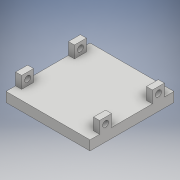
# Autodesk Inventor part: steven_example
Saved by Autodesk Inventor 2018 (Build 220112000, 112)
## iProperties
Created: 2018-03-21
Part Number: steven_example
Material: Generic
Document SubType Name: Modeling
Designer: dvyen
Density: 1 g/cm^3
Appearance: Default
Author: dvyen
Autodesk Inventor part; units mm, degrees
ref_plane "YZ Plane" through (0, 0, 0) normal (1, 0, 0) x (0, 1, 0)
ref_plane "XZ Plane" through (0, 0, 0) normal (0, 1, 0) x (-1, 0, 0)
ref_plane "XY Plane" through (0, 0, 0) normal (0, 0, 1) x (1, 0, 0)
sketch "Sketch1" plane through (0, 0, 0) normal (0, 0, 1) x (1, 0, 0)
  line L0 (-35, 35) -> (35, 35)
  line L1 (35, 35) -> (35, -35)
  line L2 (35, -35) -> (-35, -35)
  line L3 (-35, -35) -> (-35, 35)
  point P0 (0, 0)
  dimension "d0" = 70
  dimension "d1" = 70
  dimension "d2" = 35
  dimension "d3" = 35
  constraints: 8 end point, 2 parallel, 1 horizontal, 1 perpendicular
  measures "d0" distance of L0.start L0.end
  measures "d1" distance of L2.end L0.start
  measures "d2" distance from line of point (0, 0) L3
  measures "d3" distance from line of point (0, 0) L0
extrude "Extrusion1" add sketch "Sketch1" along normal blind 8
sketch "Sketch2" plane through (0, 0, 8) normal (0, 0, 1) x (1, 0, 0)
  line L0 (-35, 35) -> (-35, -35) projected
  line L1 (-35, 27) -> (-30, 27)
  line L2 (-30, 27) -> (-30, 17)
  line L3 (-30, 17) -> (-35, 17)
  line L4 (-35, 17) -> (-35, 27)
  line L5 (35, 35) -> (-35, 35) projected
  line L6 (0, -49) -> (0, 49) projected
  line L7 (35, 27) -> (30, 27)
  line L8 (30, 27) -> (30, 17)
  line L9 (30, 17) -> (35, 17)
  line L10 (35, 17) -> (35, 27)
  line L11 (-49, 0) -> (49, 0) projected
  line L12 (-35, -27) -> (-30, -27)
  line L13 (-30, -27) -> (-30, -17)
  line L14 (-30, -17) -> (-35, -17)
  line L15 (-35, -17) -> (-35, -27)
  line L16 (30, -17) -> (35, -17)
  line L17 (30, -27) -> (30, -17)
  line L18 (35, -27) -> (30, -27)
  line L19 (35, -17) -> (35, -27)
  point P0 (0, 0)
  dimension "d7" = 10
  dimension "d8" = 8
  dimension "d9" = 5
  constraints: 32 end point, 12 symmetric about line, 2 parallel, 1 horizontal, 1 perpendicular, 1 point on line
  measures "d7" distance between parallel lines of L3 L1
  measures "d8" distance between parallel lines of L5 L1
  measures "d9" distance of L1.start L1.end
extrude "Extrusion2" add sketch "Sketch2" along normal blind 10 contours L14 L13 L12 L0 | L1 L2 L3 L0 | L10 L9 L8 L7 | L16 L19 L18 L17
sketch "Sketch3" plane through (-35, -35, 0) normal (-1, 0, 0) x (0, 0, 1)
  line L0 (8, 62) -> (8, 52) projected
  line L1 (18, 62) -> (18, 52) projected
  line L2 (8, 62) -> (18, 62) projected
  line L3 (8, 52) -> (18, 52) projected
  line L4 (8, 18) -> (8, 8) projected
  line L5 (8, 18) -> (18, 18) projected
  line L6 (8, 8) -> (18, 8) projected
  line L7 (18, 18) -> (18, 8) projected
  circle A0 centre (13, 57) radius 2.5
  circle A1 centre (13, 13) radius 2.5
  point P0 (0, 35)
  dimension "d12" = 5
  dimension "d13" = 5
  dimension "d14" = 5
  dimension "d15" = 5
  dimension "d17" = 5
  constraints: 2 centre point, 1 equal radius
  measures "d12" diameter of A0
  measures "d13" distance from line of L1 A0.centre
  measures "d14" distance from line of L2 A0.centre
  measures "d15" distance from line of L7 A1.centre
  measures "d17" distance from line of L6 A1.centre
extrude "Extrusion3" cut sketch "Sketch3" against normal through all contours A0 | A1
equation "\"d1\" = d0"
equation "\"d2\" = 0.5 * d0"
equation "\"d3\" = 0.5 * d0"
equation "\"d8\" = width"
equation "\"width\" = 8"
body "Solid1"
